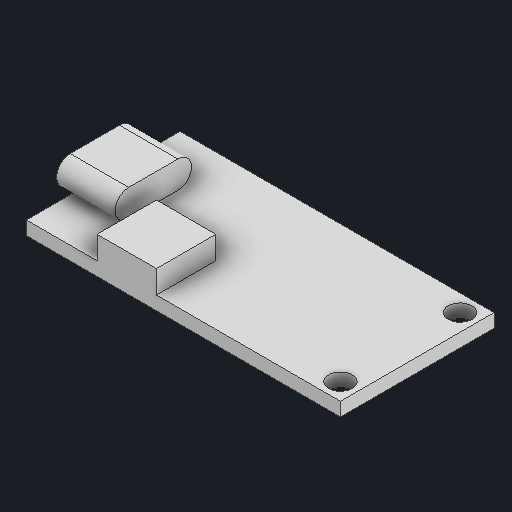
# Autodesk Inventor part: 충전모듈
Saved by Autodesk Inventor 2027.1 (Build 311270010, 270A)
## iProperties
Created: 2026-08-07
Part Number: 충전모듈
Material: 일반
Document SubType Name: Modeling
Designer: moieboy9999
Mass: 4 g
Surface Area: 17.2901 cm^2
Volume: 1.36767 cm^3
Density: 2.92468 g/cm^3
Appearance: 기본값
Author: moieboy9999
Autodesk Inventor part; units mm, degrees
ref_plane "YZ Plane" through (0, 0, 0) normal (1, 0, 0) x (0, 1, 0)
ref_plane "XZ Plane" through (0, 0, 0) normal (0, 1, 0) x (-1, 0, 0)
ref_plane "XY Plane" through (0, 0, 0) normal (0, 0, 1) x (1, 0, 0)
sketch "스케치1" plane through (0, 0, 0) normal (0, 1, 0) x (-1, 0, 0)
  line L0 (0, 0) -> (-37, 0)
  line L1 (-37, 0) -> (-37, -18.1)
  line L2 (-37, -18.1) -> (0, -18.1)
  line L3 (0, -18.1) -> (0, 0)
  dimension "d0" = 37
  dimension "d1" = 18.1
  constraints: 8 end point, 2 parallel, 1 horizontal, 1 perpendicular
  measures "d0" distance of L2.end L1.end
  measures "d1" distance of L1.end L0.end
extrude "돌출1" add sketch "스케치1" along normal blind 1.6
sketch "스케치2" plane through (0, 1.6, 0) normal (0, 1, 0) x (1, 0, 0)
  line L0 (0, 18.1) -> (0, 0) projected
  line L1 (0, 9.05) -> (0, 4.55)
  line L2 (0, 4.55) -> (5.9, 4.55)
  line L3 (5.9, 4.55) -> (5.9, 13.55)
  line L4 (5.9, 13.55) -> (0, 13.55)
  line L5 (0, 13.55) -> (0, 4.55)
  line L6 (5.9, 4.55) -> (-1, 4.55)
  line L7 (-1, 4.55) -> (-1, 13.55)
  line L8 (-1, 13.55) -> (5.9, 13.55)
  line L9 (5.9, 13.55) -> (5.9, 4.55)
  dimension "d4" = 4.5
  dimension "d5" = 5.9
  dimension "d6" = 9
  dimension "d7" = 6.9
  constraints: 18 end point, 4 parallel, 2 horizontal, 2 perpendicular, 2 point on line, 1 midpoint
  measures "d4" distance of L1.start L1.end
  measures "d5" distance of L4.end L3.end
  measures "d6" distance of L3.end L2.end
  measures "d7" distance of L7.end L8.end
extrude "돌출2" add sketch "스케치2" along normal blind 3.2 separate body
fillet "모깎기1" radius 1.6 8 edges at (2.95, 1.6, -4.55) (-0.5, 1.6, -4.55) (2.95, 4.8, -4.55) (-0.5, 4.8, -4.55) (2.95, 4.8, -13.55) (-0.5, 4.8, -13.55) (2.95, 1.6, -13.55) (-0.5, 1.6, -13.55)
sketch "스케치3" plane through (0, 1.6, 0) normal (0, 1, 0) x (1, 0, 0)
  line L0 (0, 0) -> (37, 0) projected
  line L1 (8.3193, 0) -> (15.3193, 0)
  line L2 (15.3193, 0) -> (15.3193, 7)
  line L3 (15.3193, 7) -> (8.3193, 7)
  line L4 (8.3193, 7) -> (8.3193, 0)
  dimension "d11" = 7
  dimension "d12" = 7
  constraints: 8 end point, 2 parallel, 1 horizontal, 1 perpendicular, 1 point on line
  measures "d11" distance of L3.end L2.end
  measures "d12" distance of L2.end L1.end
extrude "돌출3" add sketch "스케치3" along normal blind 2.7 separate body
combine bodies "결합1" operation type add bodies to combine 3 1 2
sketch "스케치4" plane through (8.3193, 1.6, -7) normal (0, 1, 0) x (1, 0, 0)
  line L0 (28.6807, -7) -> (28.6807, 11.1) projected
  line L1 (28.6807, -7) -> (26.6807, -7)
  line L2 (26.6807, -7) -> (26.6807, -5)
  line L3 (26.6807, -5) -> (28.6807, -5)
  line L4 (28.6807, -5) -> (28.6807, -7)
  line L5 (28.6807, 11.1) -> (-8.3193, 11.1) projected
  line L6 (28.6807, 11.1) -> (26.6807, 11.1)
  line L7 (26.6807, 11.1) -> (26.6807, 9.1)
  line L8 (26.6807, 9.1) -> (28.6807, 9.1)
  line L9 (28.6807, 9.1) -> (28.6807, 11.1)
  circle A0 centre (26.6807, -5) radius 1.4
  circle A1 centre (26.6807, 9.1) radius 1.4
  point P0 (-8.3193, -7)
  dimension "d15" = 2
  dimension "d16" = 2
  dimension "d17" = 2
  dimension "d18" = 2
  dimension "d19" = 2.8
  dimension "d20" = 2.8
  constraints: 16 end point, 4 parallel, 2 centre point, 2 coincident, 2 horizontal, 2 perpendicular
  measures "d15" distance of L2.end L3.end
  measures "d16" distance of L1.end L2.end
  measures "d17" distance of L8.end L7.end
  measures "d18" distance of L7.end L6.end
  measures "d19" diameter of A0
  measures "d20" diameter of A1
extrude "돌출4" cut sketch "스케치4" against normal blind 10 contours A0 L2 L3 | L3 L2 A0 | A1 L7 L8 | L8 L7 A1 bodies 3
